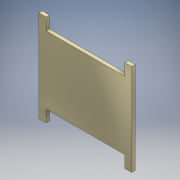
# Autodesk Inventor part: ET13
Saved by Autodesk Inventor 2016 (Build 200138000, 138)
## iProperties
Created: 2016-03-24
Part Number: ET13
Material: Genérico
Document SubType Name: Modeling
Designer: Usuario1
Density: 1 g/cm^3
Appearance: Valor por defecto
Author: Usuario1
Autodesk Inventor part; units mm, degrees
ref_plane "YZ Plane" through (0, 0, 0) normal (1, 0, 0) x (0, 1, 0)
ref_plane "XZ Plane" through (0, 0, 0) normal (0, 1, 0) x (-1, 0, 0)
sketch "Boceto1" plane through (0, 0, 0) normal (0, 1, 0) x (-1, 0, 0)
  line L0 (3.7029, -0.5193) -> (0.2952, -0.5193)
  line L1 (3.7029, -3.4471) -> (0.2952, -3.4471)
  line L2 (3.7029, -0.5193) -> (3.7029, 0)
  line L3 (3.7029, 0) -> (5.1802, 0)
  line L4 (3.7029, -3.4471) -> (3.7029, -3.9663)
  line L5 (3.7029, -3.9663) -> (5.1802, -3.9663)
  line L6 (4.0125, -3.9663) -> (4.0125, 0)
  line L7 (5.1802, -3.9663) -> (5.1802, 0)
  line L8 (0.2952, -0.5193) -> (0.2952, 0)
  line L9 (0.2952, 0) -> (0, 0)
  line L10 (0, 0) -> (-1.1677, 0)
  line L11 (-1.1677, 0) -> (-1.1677, -3.9663)
  line L12 (-1.1677, -3.9663) -> (0, -3.9663)
  line L13 (0, -3.9663) -> (0.2952, -3.9663)
  line L14 (0.2952, -3.9663) -> (0.2952, -3.4471)
  line L15 (0, 0) -> (0, -3.9663)
  line L16 (3.7029, -2.6832) -> (3.7029, -1.2832)
  line L17 (3.7029, -2.6832) -> (3.2029, -2.6832)
  line L18 (3.2029, -2.6832) -> (3.2029, -1.2832)
  line L19 (3.7029, -1.2832) -> (3.2029, -1.2832)
  line L20 (3.3553, -1.6053) -> (3.5807, -1.6053)
  line L21 (3.5807, -1.6053) -> (3.5807, -2.361)
  line L22 (3.5807, -2.361) -> (3.3553, -2.361)
  line L23 (3.3553, -2.361) -> (3.3553, -1.6053)
  circle A0 centre (3.4529, -2.9578) radius 0.1824
  line L24 (0.2952, -3.9663) -> (3.7029, -3.9663)
  line L25 (0.2952, 0) -> (3.7029, 0)
  point P0 (0, 0)
  constraints: 52 end point, 2 point on line, 1 centre point
extrude "Extrusión1" add sketch "Boceto1" along normal blind 0.15 contours L2 L3 L6 L5 L4 L1 L14 L13 L15 L9 L8 L0 | L17 L18 L19 L16 | L20 L21 L22 L23 | A0
sketch "Boceto2" plane through (0, 0.15, 0) normal (0, 1, 0) x (1, 0, 0)
  line L0 (-3.7029, 0.5193) -> (-0.2952, 0.5193)
  line L1 (-3.7029, 3.4471) -> (-0.2952, 3.4471)
  line L2 (-3.7029, 0.5193) -> (-3.7029, 0)
  line L3 (-3.7029, 0) -> (-5.1802, 0)
  line L4 (-3.7029, 3.4471) -> (-3.7029, 3.9663)
  line L5 (-3.7029, 3.9663) -> (-5.1802, 3.9663)
  line L6 (-4.0125, 3.9663) -> (-4.0125, 0)
  line L7 (-5.1802, 3.9663) -> (-5.1802, 0)
  line L8 (-0.2952, 0.5193) -> (-0.2952, 0)
  line L9 (-0.2952, 0) -> (0, 0)
  line L10 (0, 0) -> (1.1677, 0)
  line L11 (1.1677, 0) -> (1.1677, 3.9663)
  line L12 (1.1677, 3.9663) -> (0, 3.9663)
  line L13 (0, 3.9663) -> (-0.2952, 3.9663)
  line L14 (-0.2952, 3.9663) -> (-0.2952, 3.4471)
  line L15 (0, 0) -> (0, 3.9663)
  line L16 (-3.7029, 2.6832) -> (-3.7029, 1.2832)
  line L17 (-3.7029, 2.6832) -> (-3.2029, 2.6832)
  line L18 (-3.2029, 2.6832) -> (-3.2029, 1.2832)
  line L19 (-3.7029, 1.2832) -> (-3.2029, 1.2832)
  line L20 (-3.3553, 1.6053) -> (-3.5807, 1.6053)
  line L21 (-3.5807, 1.6053) -> (-3.5807, 2.361)
  line L22 (-3.5807, 2.361) -> (-3.3553, 2.361)
  line L23 (-3.3553, 2.361) -> (-3.3553, 1.6053)
  circle A0 centre (-3.4529, 2.9578) radius 0.1824
  line L24 (-0.2952, 3.9663) -> (-3.7029, 3.9663)
  line L25 (-0.2952, 0) -> (-3.7029, 0)
  line L26 (-3.7029, 0.5193) -> (-0.2952, 0.5193) projected
  line L27 (-0.2952, 0.5193) -> (-0.2952, 0) projected
  line L28 (-0.2952, 0) -> (0, 0) projected
  line L29 (0, 0) -> (0, 3.9663) projected
  line L30 (0, 3.9663) -> (-0.2952, 3.9663) projected
  line L31 (-0.2952, 3.9663) -> (-0.2952, 3.4471) projected
  line L32 (-0.2952, 3.4471) -> (-3.7029, 3.4471) projected
  line L33 (-3.7029, 3.4471) -> (-3.7029, 3.9663) projected
  line L34 (-3.7029, 3.9663) -> (-4.0125, 3.9663) projected
  line L35 (-4.0125, 3.9663) -> (-4.0125, 0) projected
  line L36 (-4.0125, 0) -> (-3.7029, 0) projected
  line L37 (-3.7029, 0) -> (-3.7029, 0.5193) projected
  point P0 (0, 0)
  constraints: 52 end point, 2 point on line, 1 centre point
extrude "Extrusión2" cut sketch "Boceto2" against normal blind 0.05 contours L17 L18 L19 L16 | L20 L21 L22 L23
sketch "Boceto3" plane through (0, 0.15, 0) normal (0, 1, 0) x (1, 0, 0)
  line L0 (-3.7029, 0.5193) -> (-0.2952, 0.5193)
  line L1 (-3.7029, 3.4471) -> (-0.2952, 3.4471)
  line L2 (-3.7029, 0.5193) -> (-3.7029, 0)
  line L3 (-3.7029, 0) -> (-5.1802, 0)
  line L4 (-3.7029, 3.4471) -> (-3.7029, 3.9663)
  line L5 (-3.7029, 3.9663) -> (-5.1802, 3.9663)
  line L6 (-4.0125, 3.9663) -> (-4.0125, 0)
  line L7 (-5.1802, 3.9663) -> (-5.1802, 0)
  line L8 (-0.2952, 0.5193) -> (-0.2952, 0)
  line L9 (-0.2952, 0) -> (0, 0)
  line L10 (0, 0) -> (1.1677, 0)
  line L11 (1.1677, 0) -> (1.1677, 3.9663)
  line L12 (1.1677, 3.9663) -> (0, 3.9663)
  line L13 (0, 3.9663) -> (-0.2952, 3.9663)
  line L14 (-0.2952, 3.9663) -> (-0.2952, 3.4471)
  line L15 (0, 0) -> (0, 3.9663)
  line L16 (-3.7029, 2.6832) -> (-3.7029, 1.2832)
  line L17 (-3.7029, 2.6832) -> (-3.2029, 2.6832)
  line L18 (-3.2029, 2.6832) -> (-3.2029, 1.2832)
  line L19 (-3.7029, 1.2832) -> (-3.2029, 1.2832)
  line L20 (-3.3553, 1.6053) -> (-3.5807, 1.6053)
  line L21 (-3.5807, 1.6053) -> (-3.5807, 2.361)
  line L22 (-3.5807, 2.361) -> (-3.3553, 2.361)
  line L23 (-3.3553, 2.361) -> (-3.3553, 1.6053)
  circle A0 centre (-3.4529, 2.9578) radius 0.1824
  line L24 (-0.2952, 3.9663) -> (-3.7029, 3.9663)
  line L25 (-0.2952, 0) -> (-3.7029, 0)
  line L26 (-3.2029, 1.2832) -> (-3.7029, 1.2832) projected
  line L27 (-3.7029, 1.2832) -> (-3.7029, 2.6832) projected
  line L28 (-3.7029, 2.6832) -> (-3.2029, 2.6832) projected
  line L29 (-3.2029, 2.6832) -> (-3.2029, 1.2832) projected
  line L30 (-3.7029, 0.5193) -> (-0.2952, 0.5193) projected
  line L31 (-0.2952, 0.5193) -> (-0.2952, 0) projected
  line L32 (-0.2952, 0) -> (0, 0) projected
  line L33 (0, 0) -> (0, 3.9663) projected
  line L34 (0, 3.9663) -> (-0.2952, 3.9663) projected
  line L35 (-0.2952, 3.9663) -> (-0.2952, 3.4471) projected
  line L36 (-0.2952, 3.4471) -> (-3.7029, 3.4471) projected
  line L37 (-3.7029, 3.4471) -> (-3.7029, 3.9663) projected
  line L38 (-3.7029, 3.9663) -> (-4.0125, 3.9663) projected
  line L39 (-4.0125, 3.9663) -> (-4.0125, 0) projected
  line L40 (-4.0125, 0) -> (-3.7029, 0) projected
  line L41 (-3.7029, 0) -> (-3.7029, 0.5193) projected
  point P0 (0, 0)
  constraints: 52 end point, 2 point on line, 1 centre point
extrude "Extrusión3" add sketch "Boceto3" along normal blind 0.25 contours A0
fillet "Empalme1" radius 0.05 1 edges at (-3.6353, 0.4, -2.9578)
ref_plane "Plano de trabajo1" through (0, 0, -2.9578) normal (0, 0, 1) x (1, 0, 0)
sketch "Boceto4" plane through (0, 0, -2.9578) normal (0, 0, 1) x (1, 0, 0)
  line L0 (-3.6353, 0.15) -> (-3.2706, 0.15) projected
  line L1 (-3.2706, 0.35) -> (-3.6353, 0.35) projected
  line L2 (-3.2706, 0.15) -> (-3.2706, 0.17)
  line L3 (-3.2706, 0.15) -> (-3.2706, 0.35) projected
  line L4 (-3.3206, 0.17) -> (-3.3206, 0.15)
  line L5 (-3.6353, 0.15) -> (-3.2706, 0.15) projected
  line L6 (-3.2706, 0.15) -> (-3.3206, 0.15)
  line L7 (-3.4529, 0.35) -> (-3.4529, 0.5679)
  line L8 (-3.3206, 0.17) -> (-3.3206, 0.19)
  line L9 (-3.3206, 0.19) -> (-3.2706, 0.19)
  line L10 (-3.2706, 0.19) -> (-3.2706, 0.15)
  point P0 (0, 0)
  dimension "d9" = 0.05
  dimension "d10" = 0.02
  constraints: 14 end point, 3 perpendicular, 3 point on line, 2 vertical, 1 collinear, 1 midpoint
  measures "d9" distance of L2.end L4.start
  measures "d10" distance of L4.start L8.end
revolve "Revolución1" cut sketch "Boceto4" angle 360 about axis through (-3.4529, 0.35, -2.9578) along (0, 1, 0)
ref_plane "Plano de trabajo2" through (0, 0, -2.5578) normal (0, 0, 1) x (1, 0, 0)
sketch "Boceto5" plane through (0, 0, -2.5578) normal (0, 0, 1) x (1, 0, 0)
  line L0 (-3.2706, 0.19) -> (-3.6353, 0.19) projected
  line L1 (-3.2706, 0.35) -> (-3.6353, 0.35) projected
  line L2 (-3.6353, 0.19) -> (-3.6353, 0.35) projected
  line L3 (-3.2706, 0.35) -> (-3.6353, 0.35) projected
  line L4 (-3.3206, 0.19) -> (-3.5853, 0.19) projected
  line L5 (-3.2706, 0.19) -> (-3.2706, 0.35) projected
  circle A0 centre (-3.4529, 0.27) radius 0.05
  point P0 (0, 0)
  dimension "d13" = 0.1
  constraints: 1 centre point
  measures "d13" diameter of A0
extrude "Extrusión4" cut sketch "Boceto5" against normal blind 25 contours A0
sketch "Boceto6" plane through (0, 0, 0) normal (1, 0, 0) x (0, 1, 0)
  line L0 (0.35, -3.1402) -> (0.35, -2.7755) projected
  line L1 (0.19, -2.7755) -> (0.35, -2.7755) projected
  line L2 (0.19, -3.0902) -> (0.19, -2.8254) projected
  circle A0 centre (0.27, -2.9578) radius 0.05
  point P0 (0, 0)
  dimension "d16" = 0.1
  constraints: 1 centre point
  measures "d16" diameter of A0
extrude "Extrusión5" cut sketch "Boceto6" against normal blind 25
